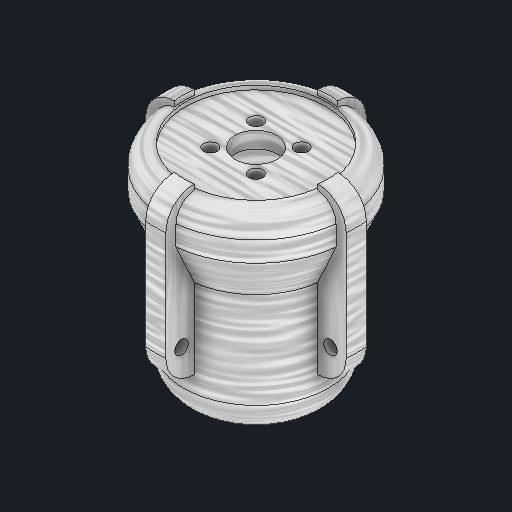
# Autodesk Inventor part: Corredor
Saved by Autodesk Inventor 2025.4 (Build 294407000, 407)
## iProperties
Created: 2024-11-15
Part Number: Corredor
Material: Aluminum 7075
Document SubType Name: Modeling
Designer: j.santaa
Density: 2.81 g/cm^3
Appearance: Satin - Brushed Heavy
Mass: 86.0623 g
Surface Area: 155.469 cm^2
Volume: 30.6272 cm^3
Author: j.santaa
Autodesk Inventor part; units mm, degrees
ref_plane "YZ Plane" through (0, 0, 0) normal (1, 0, 0) x (0, 1, 0)
sketch "Sketch4" plane through (0, 0, 0) normal (1, 0, 0) x (0, 1, 0)
  line L0 (5.2, 0) -> (15, 0)
  line L1 (15, 0) -> (15, -45)
  line L2 (0, 5) -> (0, -45)
  line L3 (5.2, 0) -> (5.2, 5)
  line L4 (5.2, 5) -> (22.5, 5)
  line L5 (22.5, 5) -> (22.5, -5)
  line L6 (22.5, -5) -> (18, -14.9216)
  line L7 (18, -14.9216) -> (18, -45)
  line L8 (18, -45) -> (15, -45)
  point P0 (0, 0)
  point P1 (19.25, -5)
  dimension "d11" = 30
  dimension "d12" = 10.4
  dimension "d13" = 5
  dimension "d14" = 10
  dimension "d15" = 45
  dimension "d18" = 3.25
  dimension "d19" = 10
  dimension "d59" = 50
  dimension "d84" = 3
  constraints: 18 end point, 4 horizontal alignment, 4 vertical, 2 perpendicular, 1 horizontal, 1 point on line
  measures "d11" diameter of L1 L2
  measures "d12" diameter of L3 L2
  measures "d13" distance of L0.start L3.end
  measures "d14" distance of L4.end L5.end
  measures "d15" diameter of L5 L2
  measures "d18" distance of L5.end point (19.25, -5)
  measures "d19" distance of L6.end point (19.25, -5)
  measures "d59" distance between parallel lines of L8 L4
  measures "d84" distance of L7.end L1.end
revolve "Revolution2" add sketch "Sketch4" angle 360 about axis through (0, 0, 5) along (0, 0, -1)
ref_plane "Work Plane1" through (0, 0, -19.682) normal (0, 0, 1) x (1, 0, 0)
sketch "Sketch5" plane through (0, 0, -19.682) normal (0, 0, 1) x (1, 0, 0)
  arc A0 (-24.8747, 2.5) -> (-24.8747, -2.5) centre (0, 0) ccw
  line L0 (-24.8747, 2.5) -> (-17.8255, 2.5)
  line L1 (-24.8747, -2.5) -> (-17.8255, -2.5)
  circle A1 centre (0, 0) radius 18 projected
  point P0 (-25, 0)
  point P1 (-18, 0)
  dimension "Dedos" = 5
  dimension "d72" = 7
  constraints: 6 point on circle, 4 end point, 2 horizontal alignment, 1 centre point, 1 coincident, 1 concentric, 1 horizontal, 1 parallel
  measures "Dedos" distance between parallel lines of L1 L0
  measures "d72" distance of point (-25, 0) point (-18, 0)
extrude "Extrusion1" add sketch "Sketch5" against normal blind 15 contours L0 A1 L1 A0
ref_plane "Work Plane2" through (-24.8747, 0, -19.682) normal (0, -1, 0) x (1, 0, 0)
sketch "Sketch7" plane through (-24.8747, 0, -19.682) normal (0, -1, 0) x (1, 0, 0)
  line L0 (-0.1253, 0) -> (-0.1253, -15) projected
  circle A0 centre (-0.8653, -7.5) radius 1.5
  line L1 (6.8747, -25.318) -> (42.8747, -25.318) projected
  line L2 (24.8747, -25.318) -> (24.8747, 24.682) construction
  line L3 (19.6747, 24.682) -> (30.0747, 24.682) projected
  point P0 (24.8747, 19.682)
  point P1 (-0.1253, -7.5)
  dimension "d45" = 3
  dimension "d83" = 25.74
  constraints: 3 midpoint, 2 end point, 1 centre point, 1 coincident, 1 horizontal alignment
  measures "d45" diameter of A0
  measures "d83" distance from line of L2 A0.centre
fillet "Fillet2" radius 7 1 edges at (-25, 0, -34.682)
pattern_circular "Circular Pattern1" count 4 over 360 about axis through (0, 0, -29.9608) along (0, 0, -1) of "Extrusion1", "Fillet2"
fillet "Fillet3" radius 8 1 edges at (0, -18, -45)
fillet "Fillet3" radius 5 1 edges at (0, -22.5, 5)
sketch "Sketch8" plane through (0, 0, 5) normal (0, 0, 1) x (1, 0, 0)
  line L0 (-5.657, -5.657) -> (5.657, -5.657) construction
  line L1 (5.657, -5.657) -> (5.657, 5.657) construction
  line L2 (5.657, 5.657) -> (-5.657, 5.657) construction
  line L3 (-5.657, 5.657) -> (-5.657, -5.657) construction
  line L4 (-5.657, -5.657) -> (5.657, 5.657) construction
  line L5 (5.657, -5.657) -> (-5.657, 5.657) construction
  point P0 (0, 0)
  dimension "d51" = 11.314
  constraints: 12 end point, 4 coincident, 2 midpoint, 2 parallel, 2 perpendicular, 1 horizontal
  measures "d51" distance of L2.end L0.start
hole "Hole2" at (-5.657, -5.657, 5) at (-5.657, 5.657, 5) at (5.657, 5.657, 5) at (5.657, -5.657, 5) direction (0, 0, -1) diameter 3.4 end through all clearance for "Countersunk Flat Head Screw ISO 2009/7046" size "M3" standard "ISO"
sketch "Boceto10" plane through (2.5, -17.8255, -19.682) normal (0, 0, 1) x (0, -1, 0)
  line L0 (7.0491, 0) -> (0, 0) projected
  arc A0 (0, -5) -> (0, 0) centre (-17.8255, -2.5) ccw projected
  line L1 (0, -5) -> (7.0491, -5) projected
  arc A1 (7.0491, -5) -> (7.0491, 0) centre (-17.8255, -2.5) ccw projected
  point P0 (-17.8255, -2.5)
extrude "Extrusión3" add sketch "Boceto10" along normal blind 26
fillet "Empalme4" radius 7 1 edges at (0, -25, 6.318)
pattern_circular "Patrón circular2" count 4 over 360 about axis through (0, 0, -29.9608) along (0, 0, -1) of "Empalme4", "Extrusión3"
sketch "Boceto11" plane through (0, 0, 5) normal (0, 0, 1) x (-1, 0, 0)
  circle A0 centre (0, 0) radius 17.5 projected
  circle A1 centre (0, 0) radius 5.2 projected
  circle A2 centre (5.657, 5.657) radius 1.7 projected
  circle A3 centre (5.657, -5.657) radius 1.7 projected
  circle A4 centre (-5.657, -5.657) radius 1.7 projected
  circle A5 centre (-5.657, 5.657) radius 1.7 projected
  point P0 (0, 0)
extrude "Extrusión4" cut sketch "Boceto11" against normal blind 1
sketch "Boceto12" plane through (-17.8255, 2.5, -14.9216) normal (0, 1, 0) x (1, 0, 0)
  line L0 (32.8255, 30.0784) -> (2.8255, 30.0784) projected
  line L1 (12.6255, -18.9216) -> (23.0255, -18.9216) projected
  line L2 (17.8255, -18.9216) -> (17.8255, 30.0784) construction
  point P0 (-3.1745, 12.2604)
  dimension "d85" = 17.818
  dimension "d86" = 21
  constraints: 2 end point, 2 midpoint
  measures "d85" distance from line of L0 point (-3.174, 12.26)
  measures "d86" distance from line of L2 point (-3.174, 12.26)
hole "Agujero3" at (-21, 2.5, -27.182) direction (0, -1, 0) diameter 3.4 end through all clearance for "Tornillo de cabeza plana avellanada ISO 2009/7046" size "M3" standard "ISO"
pattern_circular "Patrón circular3" count 4 over 360 about axis through (0, 0, -29.9608) along (0, 0, -1) of "Agujero3"
body "Solid2"
